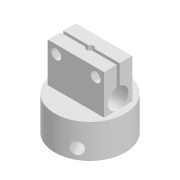
# Autodesk Inventor part: 20_Cube_Insert_Lightsheet_FEPTube_Rotating_hollomotor_v1
Saved by Autodesk Inventor 2022 (Build 260153000, 153)
## iProperties
Created: 2022-03-03
Part Number: 20_Cube_Insert_Lightsheet_FEPTube_Rotating_hollomotor_v1
Material: Generic
Document SubType Name: Modeling
Designer: Prakash Lab
Density: 1 g/cm^3
Appearance: Default
Author: Prakash Lab
Autodesk Inventor part; units mm, degrees
ref_plane "YZ Plane" through (0, 0, 0) normal (1, 0, 0) x (0, 1, 0)
ref_plane "XZ Plane" through (0, 0, 0) normal (0, 1, 0) x (-1, 0, 0)
ref_plane "XY Plane" through (0, 0, 0) normal (0, 0, 1) x (1, 0, 0)
sketch "Sketch14" plane through (0, 0, 0) normal (0, 1, 0) x (-1, 0, 0)
  circle A0 centre (0, 0) radius 2.45
  circle A1 centre (0, 0) radius 12.5
  dimension "d69" = 4.9
  dimension "d70" = 25
  constraints: 2 centre point, 2 coincident
  measures "d69" diameter of A0
  measures "d70" diameter of A1
extrude "Extrusion9" add sketch "Sketch14" along normal blind 12
sketch "Sketch15" plane through (0, 0, 0) normal (1, 0, 0) x (0, 1, 0)
  circle A0 centre (3.6206, 0) radius 2.058
  point P0 (0, 0)
  constraints: 1 centre point
extrude "Extrusion10" cut sketch "Sketch15" against normal blind 15
pattern_circular "Circular Pattern2" count 3 over 360 about axis through (0, 0, 0) along (0, 1, 0) of "Extrusion10"
sketch "Sketch16" plane through (0, 0, 0) normal (1, 0, 0) x (0, 1, 0)
  line L0 (12, -12.5) -> (12, 12.5) projected
  line L1 (26, -5) -> (12, -5)
  line L2 (12, -5) -> (12, 5)
  line L3 (12, 5) -> (26, 5)
  line L4 (26, 5) -> (26, -5)
  line L5 (26, -5) -> (12, 5) construction
  line L6 (12, -5) -> (26, 5) construction
  point P0 (0, 0)
  point P1 (19, 0)
  dimension "d78" = 10
  dimension "d81" = 14
  constraints: 12 end point, 2 midpoint, 2 parallel, 1 horizontal, 1 perpendicular, 1 point on line
  measures "d78" distance of L1.end L2.end
  measures "d81" distance between parallel lines of L0 L4
extrude "Extrusion11" add sketch "Sketch16" along normal mid plane 20
sketch "Sketch17" plane through (10, 0, 0) normal (1, 0, 0) x (0, 0, -1)
  line L0 (0.5, 15.4327) -> (-0.5, 15.4327)
  line L1 (-0.5, 15.4327) -> (-0.5, 27.4327)
  line L2 (-0.5, 27.4327) -> (0.5, 27.4327)
  line L3 (0.5, 27.4327) -> (0.5, 15.4327)
  line L4 (0.5, 15.4327) -> (-0.5, 27.4327) construction
  line L5 (-0.5, 15.4327) -> (0.5, 27.4327) construction
  circle A0 centre (0, 15.4327) radius 3.6334
  point P0 (0, 0)
  point P1 (0, 21.4327)
  point P2 (-0.5, 19.0315)
  point P3 (0.5, 19.0315)
  dimension "d82" = 1
  dimension "d83" = 12
  constraints: 12 end point, 3 midpoint, 2 parallel, 1 centre point, 1 horizontal, 1 perpendicular
  measures "d82" distance between parallel lines of L3 L1
  measures "d83" distance between parallel lines of L2 L0
extrude "Extrusion12" cut sketch "Sketch17" against normal through all
sketch "Sketch18" plane through (-10, 12, 5) normal (0, 0, 1) x (1, 0, 0)
  line L0 (20, 0) -> (0, 0) projected
  line L1 (20, 14) -> (20, 0) projected
  line L2 (20, 14) -> (0, 14) projected
  line L3 (0, 0) -> (0, 14) projected
  line L4 (3, 11) -> (17, 11)
  line L5 (17, 11) -> (17, 3)
  line L6 (17, 3) -> (3, 3)
  line L7 (3, 3) -> (3, 11)
  point P0 (10, -12)
  dimension "d86" = 3
  constraints: 8 end point, 3 other
  measures "d86" distance between parallel lines of L2 L4
hole "Hole1" at (-7, 23, 5) at (7, 23, 5) direction (0, 0, -1) diameter 3.5 depth 5.5 tip angle 118
sketch "Sketch19" plane through (10, 26, -5) normal (0, 0, -1) x (-1, 0, 0)
  circle A0 centre (3, -3) radius 1.75 projected
  circle A1 centre (17, -3) radius 1.75 projected
  point P0 (10, -26)
  point P1 (2.1717, -1.4585)
  point P2 (3.8283, -1.4585)
  point P3 (16.1717, -1.4585)
  point P4 (17.8283, -1.4585)
hole "Hole2" at (7, 23, -5) at (-7, 23, -5) direction (0, 0, 1) diameter 2.8 end through all
sketch "Sketch20" plane through (-10, 26, 5) normal (0, 1, 0) x (1, 0, 0)
  circle A0 centre (10, 5) radius 1.25
  point P0 (10, 5)
  point P1 (10, 7.45)
  dimension "d101" = 2.5
  constraints: 1 centre point, 1 coincident, 1 other
  measures "d101" diameter of A0
extrude "Extrusion13" cut sketch "Sketch20" against normal through all
body "Solid2"
